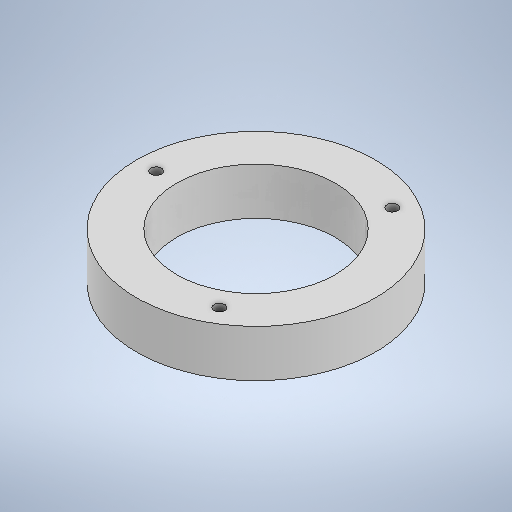
# Autodesk Inventor part: Adapter
Saved by Autodesk Inventor 2026.2 (Build 302298000, 298)
## iProperties
Created: 2026-03-06
Part Number: Adapter
Material: Generic
Document SubType Name: Modeling
Designer: mumin
Density: 1 g/cm^3
Appearance: Default
Author: mumin
Autodesk Inventor part; units mm, degrees
ref_plane "YZ Plane" through (0, 0, 0) normal (1, 0, 0) x (0, 1, 0)
ref_plane "XZ Plane" through (0, 0, 0) normal (0, 1, 0) x (-1, 0, 0)
ref_plane "XY Plane" through (0, 0, 0) normal (0, 0, 1) x (1, 0, 0)
sketch "Sketch1" plane through (0, 0, 0) normal (0, 1, 0) x (-1, 0, 0)
  circle A0 centre (0, 0) radius 40.5
  circle A1 centre (0, 0) radius 61
  dimension "d0" = 81
  dimension "d1" = 122
  constraints: 2 centre point, 2 coincident
  measures "d0" diameter of A0
  measures "d1" diameter of A1
extrude "Extrusion1" add sketch "Sketch1" along normal blind 24
sketch "Sketch2" plane through (0, 24, 0) normal (0, 1, 0) x (1, 0, 0)
  circle A0 centre (0, 0) radius 51 construction
  point P0 (-51, 0)
  point P1 (25.5, -44.1673)
  point P2 (25.5, 44.1673)
  dimension "d4" = 102
  dimension "d7" = 360
  constraints: 1 coincident, 1 horizontal alignment, 6 other
hole "Hole1" at (-51, 24, 0) at (25.5, 24, 44.1673) at (25.5, 24, -44.1673) direction (0, -1, 0) diameter 5.5 end through all
body "Solid1"
